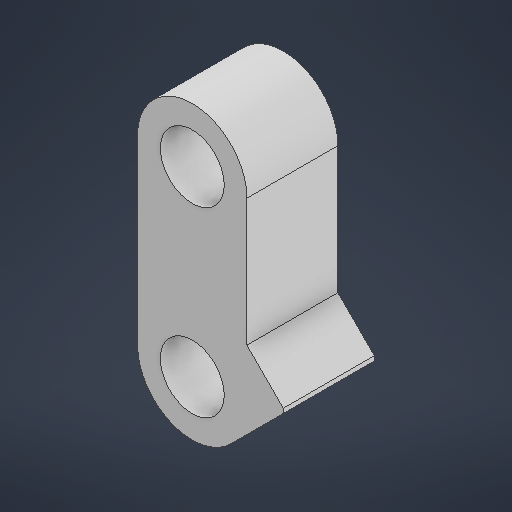
# Autodesk Inventor part: mellemStykke
Saved by Autodesk Inventor 2026.3 (Build 303398000, 398)
## iProperties
Created: 2026-05-05
Part Number: mellemStykke
Material: Generic
Document SubType Name: Modeling
Designer: frede
Density: 1 g/cm^3
Appearance: Default
Author: frede
Autodesk Inventor part; units mm, degrees
ref_plane "YZ Plane" through (0, 0, 0) normal (1, 0, 0) x (0, 1, 0)
ref_plane "XZ Plane" through (0, 0, 0) normal (0, 1, 0) x (-1, 0, 0)
ref_plane "XY Plane" through (0, 0, 0) normal (0, 0, 1) x (1, 0, 0)
sketch "Sketch1" plane through (0, 0, 0) normal (0, 0, 1) x (1, 0, 0)
  circle A0 centre (0, 0) radius 1.75
  circle A1 centre (0, -10) radius 1.75
  arc A2 (-3, -10) -> (3, -10) centre (0, -10) ccw
  arc A3 (3, 0) -> (-3, 0) centre (0, 0) ccw
  line L0 (-3, -10) -> (-3, 0)
  line L1 (3, -10) -> (3, 0)
  line L2 (2.1213, -12.1213) -> (5, -9.2426)
  line L3 (2.1213, -12.1213) -> (4.3055, -12.1213) construction
  line L4 (5, -9.2426) -> (5, -8.9926)
  line L5 (5, -8.9926) -> (3, -6.9926)
  point P0 (3, -7.757)
  dimension "d0" = 3.5
  dimension "d1" = 3.5
  dimension "d2" = 6
  dimension "d3" = 6
  dimension "d6" = 45
  dimension "d10" = 5
  dimension "d11" = 0.25
  dimension "d12" = 135
  constraints: 12 end point, 5 point on circle, 4 centre point, 3 coincident, 3 tangent, 2 point on line, 2 vertical, 1 horizontal
  measures "d0" diameter of A0
  measures "d1" diameter of A1
  measures "d2" diameter of A2
  measures "d3" diameter of A3
  measures "d6" angle of L3 L2
  measures "d10" horizontal distance of L2.end A1.centre
  measures "d11" distance of L2.end L4.end
  measures "d12" angle of L5 L4
extrude "Extrusion1" add sketch "Sketch1" along normal blind 5
body "Solid1"
